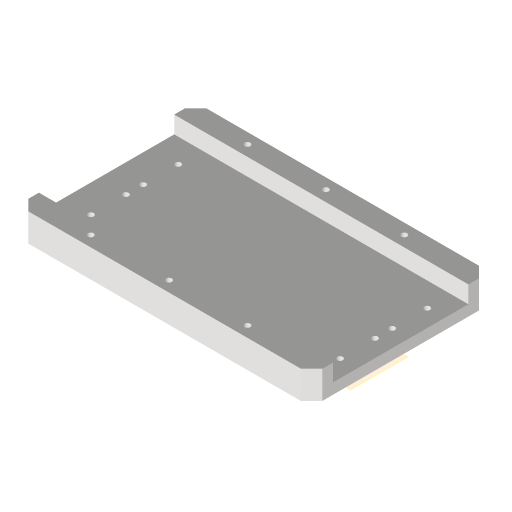
# Autodesk Inventor part: 60_Planktoscope_Wallboxmoutingplate
Saved by Autodesk Inventor 2024.1 (Build 281209000, 209)
## iProperties
Created: 2024-03-15
Part Number: 60_Planktoscope_Wallboxmoutingplate
Material: Generisch
Document SubType Name: Modeling
Designer: diederichbenedict
Density: 1 g/cm^3
Appearance: Vorgabe
Author: diederichbenedict
Autodesk Inventor part; units mm, degrees
ref_plane "YZ Plane" through (0, 0, 0) normal (1, 0, 0) x (0, 1, 0)
ref_plane "XZ Plane" through (0, 0, 0) normal (0, 1, 0) x (-1, 0, 0)
ref_plane "XY Plane" through (0, 0, 0) normal (0, 0, 1) x (1, 0, 0)
ref_plane "Arbeitsebene1" through (0, -48.6, 0) normal (0, 0, 1) x (1, 0, 0)
sketch "Skizze1" plane through (0, -48.6, 0) normal (0, 0, 1) x (1, 0, 0)
  circle A0 centre (124, 28.3) radius 1.4 projected
  circle A1 centre (124, 44.6) radius 1.4 projected
  circle A2 centre (8, 28.3) radius 1.4 projected
  circle A3 centre (8, 44.6) radius 1.4 projected
  spline S0 degree 2 poles (11.2125, 42.0174) (10.5764, 41.5903) (9.8857, 40.1908) (9.8857, 39.2184) knots 0 0 0 1 2 2 2 construction
  spline S1 degree 2 poles (14.1568, 42.7535) (13.1936, 42.7535) (11.785, 42.3991) (11.2125, 42.0174) knots 0 0 0 1 2 2 2 construction
  line L0 (18.5098, 42.7535) -> (14.1568, 42.7535) construction
  line L1 (18.5098, 31.5395) -> (18.5098, 42.7535) construction
  line L2 (15.6926, 31.5395) -> (18.5098, 31.5395) construction
  line L3 (15.6926, 35.2108) -> (15.6926, 31.5395) construction
  line L4 (14.2205, 35.2108) -> (15.6926, 35.2108) construction
  spline S2 degree 2 poles (12.2303, 35.5834) (12.6483, 35.4108) (13.6207, 35.2108) (14.2205, 35.2108) knots 0 0 0 1 2 2 2 construction
  spline S3 degree 2 poles (10.849, 36.5467) (11.1307, 36.2468) (11.8213, 35.7561) (12.2303, 35.5834) knots 0 0 0 1 2 2 2 construction
  spline S4 degree 2 poles (9.8857, 39.2184) (9.8857, 38.4369) (10.3855, 37.0193) (10.849, 36.5467) knots 0 0 0 1 2 2 2 construction
  spline S5 degree 2 poles (25.6162, 42.9898) (23.0899, 42.9898) (20.1819, 39.8637) (20.1819, 37.1465) knots 0 0 0 1 2 2 2 construction
  spline S6 degree 2 poles (31.0415, 37.1465) (31.0415, 39.8455) (28.1516, 42.9898) (25.6162, 42.9898) knots 0 0 0 1 2 2 2 construction
  spline S7 degree 2 poles (25.6162, 31.3032) (28.1516, 31.3032) (31.0415, 34.4566) (31.0415, 37.1465) knots 0 0 0 1 2 2 2 construction
  spline S8 degree 2 poles (20.1819, 37.1465) (20.1819, 34.4202) (23.0899, 31.3032) (25.6162, 31.3032) knots 0 0 0 1 2 2 2 construction
  spline S9 degree 2 poles (37.4936, 42.9898) (34.9673, 42.9898) (32.0593, 39.8637) (32.0593, 37.1465) knots 0 0 0 1 2 2 2 construction
  spline S10 degree 2 poles (42.9188, 37.1465) (42.9188, 39.8455) (40.029, 42.9898) (37.4936, 42.9898) knots 0 0 0 1 2 2 2 construction
  spline S11 degree 2 poles (37.4936, 31.3032) (40.029, 31.3032) (42.9188, 34.4566) (42.9188, 37.1465) knots 0 0 0 1 2 2 2 construction
  spline S12 degree 2 poles (32.0593, 37.1465) (32.0593, 34.4202) (34.9673, 31.3032) (37.4936, 31.3032) knots 0 0 0 1 2 2 2 construction
  line L5 (56.2684, 35.8379) -> (53.1696, 31.5395) construction
  line L6 (53.2059, 40) -> (56.2684, 35.8379) construction
  line L7 (56.2321, 40) -> (53.2059, 40) construction
  line L8 (57.8224, 37.619) -> (56.2321, 40) construction
  line L9 (59.4036, 40) -> (57.8224, 37.619) construction
  line L10 (62.4934, 40) -> (59.4036, 40) construction
  line L11 (59.4309, 35.7743) -> (62.4934, 40) construction
  line L12 (62.5479, 31.5395) -> (59.4309, 35.7743) construction
  line L13 (59.5217, 31.5395) -> (62.5479, 31.5395) construction
  line L14 (57.8678, 33.9659) -> (59.5217, 31.5395) construction
  line L15 (56.2593, 31.5395) -> (57.8678, 33.9659) construction
  line L16 (53.1696, 31.5395) -> (56.2593, 31.5395) construction
  spline S13 degree 2 poles (72.6805, 31.6667) (73.1712, 31.5031) (74.0072, 31.3396) (74.6797, 31.3396) knots 0 0 0 1 2 2 2 construction
  spline S14 degree 2 poles (71.1901, 32.3028) (71.5627, 32.1302) (72.217, 31.8121) (72.6805, 31.6667) knots 0 0 0 1 2 2 2 construction
  line L17 (71.1901, 34.084) -> (71.1901, 32.3028) construction
  line L18 (71.2992, 34.084) -> (71.1901, 34.084) construction
  spline S15 degree 2 poles (72.4896, 33.1843) (72.0807, 33.4206) (71.4718, 33.9113) (71.2992, 34.084) knots 0 0 0 1 2 2 2 construction
  spline S16 degree 2 poles (74.6615, 32.63) (74.0163, 32.63) (72.9167, 32.9481) (72.4896, 33.1843) knots 0 0 0 1 2 2 2 construction
  spline S17 degree 2 poles (77.1061, 33.7478) (76.6335, 33.1934) (75.3704, 32.63) (74.6615, 32.63) knots 0 0 0 1 2 2 2 construction
  spline S18 degree 2 poles (78.1421, 37.1374) (78.1421, 35.9833) (77.5877, 34.3203) (77.1061, 33.7478) knots 0 0 0 1 2 2 2 construction
  spline S19 degree 2 poles (77.1424, 40.527) (77.615, 39.9545) (78.1421, 38.2188) (78.1421, 37.1374) knots 0 0 0 1 2 2 2 construction
  spline S20 degree 2 poles (74.6615, 41.6812) (75.3795, 41.6812) (76.6608, 41.0905) (77.1424, 40.527) knots 0 0 0 1 2 2 2 construction
  spline S21 degree 2 poles (72.5714, 41.145) (72.9985, 41.3813) (74.0072, 41.6812) (74.6615, 41.6812) knots 0 0 0 1 2 2 2 construction
  spline S22 degree 2 poles (71.3083, 40.209) (71.5082, 40.3907) (72.1261, 40.8996) (72.5714, 41.145) knots 0 0 0 1 2 2 2 construction
  line L19 (71.1901, 40.209) -> (71.3083, 40.209) construction
  line L20 (71.1901, 42.0083) -> (71.1901, 40.209) construction
  spline S23 degree 2 poles (72.6805, 42.6626) (72.317, 42.5445) (71.5627, 42.2082) (71.1901, 42.0083) knots 0 0 0 1 2 2 2 construction
  spline S24 degree 2 poles (74.6525, 42.9534) (74.089, 42.9534) (73.0985, 42.7898) (72.6805, 42.6626) knots 0 0 0 1 2 2 2 construction
  spline S25 degree 2 poles (78.2966, 41.4085) (77.6241, 42.1628) (75.7884, 42.9534) (74.6525, 42.9534) knots 0 0 0 1 2 2 2 construction
  spline S26 degree 2 poles (79.696, 37.1374) (79.696, 38.546) (78.9781, 40.6361) (78.2966, 41.4085) knots 0 0 0 1 2 2 2 construction
  spline S27 degree 2 poles (78.2875, 32.8117) (78.9599, 33.5387) (79.696, 35.7198) (79.696, 37.1374) knots 0 0 0 1 2 2 2 construction
  spline S28 degree 2 poles (74.6797, 31.3396) (75.7702, 31.3396) (77.615, 32.0757) (78.2875, 32.8117) knots 0 0 0 1 2 2 2 construction
  line L21 (91.2735, 37.0011) -> (91.2735, 31.5395) construction
  spline S29 degree 2 poles (93.9089, 40.1908) (92.673, 40.1908) (91.2735, 38.5551) (91.2735, 37.0011) knots 0 0 0 1 2 2 2 construction
  spline S30 degree 2 poles (96.4625, 39.0185) (95.8264, 39.591) (94.5996, 40.1908) (93.9089, 40.1908) knots 0 0 0 1 2 2 2 construction
  line L22 (96.4625, 39.9545) -> (96.4625, 39.0185) construction
  line L23 (97.8802, 39.9545) -> (96.4625, 39.9545) construction
  line L24 (97.8802, 31.5395) -> (97.8802, 39.9545) construction
  line L25 (96.4625, 31.5395) -> (97.8802, 31.5395) construction
  line L26 (96.4625, 37.8281) -> (96.4625, 31.5395) construction
  spline S31 degree 2 poles (94.2815, 38.8459) (94.8086, 38.8459) (95.9263, 38.2824) (96.4625, 37.8281) knots 0 0 0 1 2 2 2 construction
  spline S32 degree 2 poles (92.9638, 38.2188) (93.1365, 38.5369) (93.7544, 38.8459) (94.2815, 38.8459) knots 0 0 0 1 2 2 2 construction
  spline S33 degree 2 poles (92.6912, 36.3377) (92.6912, 36.9193) (92.8002, 37.9189) (92.9638, 38.2188) knots 0 0 0 1 2 2 2 construction
  line L27 (92.6912, 31.5395) -> (92.6912, 36.3377) construction
  line L28 (91.2735, 31.5395) -> (92.6912, 31.5395) construction
  spline S34 degree 2 poles (100.7518, 31.5849) (101.1608, 31.4668) (101.8332, 31.3487) (102.3421, 31.3487) knots 0 0 0 1 2 2 2 construction
  spline S35 degree 2 poles (99.4705, 32.0575) (99.7158, 31.9575) (100.461, 31.6667) (100.7518, 31.5849) knots 0 0 0 1 2 2 2 construction
  line L29 (99.4705, 33.6024) -> (99.4705, 32.0575) construction
  line L30 (99.5523, 33.6024) -> (99.4705, 33.6024) construction
  spline S36 degree 2 poles (100.6337, 32.9571) (100.252, 33.1389) (99.7249, 33.457) (99.5523, 33.6024) knots 0 0 0 1 2 2 2 construction
  spline S37 degree 2 poles (102.3603, 32.5846) (101.8968, 32.5846) (100.9972, 32.7936) (100.6337, 32.9571) knots 0 0 0 1 2 2 2 construction
  spline S38 degree 2 poles (105.1411, 35.6016) (105.1411, 34.1385) (103.6689, 32.5846) (102.3603, 32.5846) knots 0 0 0 1 2 2 2 construction
  line L31 (99.316, 35.6016) -> (105.1411, 35.6016) construction
  line L32 (99.316, 36.3741) -> (99.316, 35.6016) construction
  spline S39 degree 2 poles (100.252, 39.2548) (99.7976, 38.7732) (99.316, 37.3828) (99.316, 36.3741) knots 0 0 0 1 2 2 2 construction
  spline S40 degree 2 poles (102.6875, 40.1908) (101.9059, 40.1908) (100.6973, 39.7364) (100.252, 39.2548) knots 0 0 0 1 2 2 2 construction
  spline S41 degree 2 poles (106.5769, 35.7016) (106.5769, 37.7554) (104.4232, 40.1908) (102.6875, 40.1908) knots 0 0 0 1 2 2 2 construction
  spline S42 degree 2 poles (102.3421, 31.3487) (104.3596, 31.3487) (106.5769, 33.6114) (106.5769, 35.7016) knots 0 0 0 1 2 2 2 construction
  spline S43 degree 2 poles (110.53, 40.1908) (109.0851, 40.1908) (107.4675, 37.9008) (107.4675, 35.9742) knots 0 0 0 1 2 2 2 construction
  spline S44 degree 2 poles (113.1018, 39.073) (112.5747, 39.5547) (111.2843, 40.1908) (110.53, 40.1908) knots 0 0 0 1 2 2 2 construction
  line L33 (113.1018, 39.9545) -> (113.1018, 39.073) construction
  line L34 (114.5194, 39.9545) -> (113.1018, 39.9545) construction
  line L35 (114.5194, 28.4406) -> (114.5194, 39.9545) construction
  line L36 (113.1018, 28.4406) -> (114.5194, 28.4406) construction
  line L37 (113.1018, 31.9666) -> (113.1018, 28.4406) construction
  spline S45 degree 2 poles (111.0116, 31.3759) (111.6387, 31.3759) (112.6019, 31.6667) (113.1018, 31.9666) knots 0 0 0 1 2 2 2 construction
  spline S46 degree 2 poles (107.4675, 35.9742) (107.4675, 33.8659) (109.4758, 31.3759) (111.0116, 31.3759) knots 0 0 0 1 2 2 2 construction
  spline S47 degree 2 poles (119.7266, 40.1908) (118.0181, 40.1908) (115.9734, 37.8644) (115.9734, 35.747) knots 0 0 0 1 2 2 2 construction
  spline S48 degree 2 poles (123.4888, 35.747) (123.4888, 37.8553) (121.4168, 40.1908) (119.7266, 40.1908) knots 0 0 0 1 2 2 2 construction
  spline S49 degree 2 poles (119.7266, 31.3032) (121.4805, 31.3032) (123.4888, 33.6932) (123.4888, 35.747) knots 0 0 0 1 2 2 2 construction
  spline S50 degree 2 poles (115.9734, 35.747) (115.9734, 33.6205) (118.0181, 31.3032) (119.7266, 31.3032) knots 0 0 0 1 2 2 2 construction
  spline S51 degree 2 poles (82.2678, 32.3392) (82.804, 31.8121) (84.2216, 31.3032) (85.2576, 31.3032) knots 0 0 0 1 2 2 2 construction
  spline S52 degree 2 poles (81.1955, 35.7561) (81.1955, 34.5838) (81.668, 32.9117) (82.2678, 32.3392) knots 0 0 0 1 2 2 2 construction
  line L38 (81.1955, 42.7535) -> (81.1955, 35.7561) construction
  line L39 (82.6858, 42.7535) -> (81.1955, 42.7535) construction
  line L40 (82.6858, 35.7198) -> (82.6858, 42.7535) construction
  spline S53 degree 2 poles (83.1675, 33.4933) (82.8858, 33.9204) (82.6858, 34.9655) (82.6858, 35.7198) knots 0 0 0 1 2 2 2 construction
  spline S54 degree 2 poles (85.2576, 32.5755) (84.5579, 32.5755) (83.4674, 33.0389) (83.1675, 33.4933) knots 0 0 0 1 2 2 2 construction
  spline S55 degree 2 poles (87.3386, 33.4933) (87.0388, 33.0389) (86.0028, 32.5755) (85.2576, 32.5755) knots 0 0 0 1 2 2 2 construction
  spline S56 degree 2 poles (87.8203, 35.7561) (87.8203, 34.9746) (87.6204, 33.9204) (87.3386, 33.4933) knots 0 0 0 1 2 2 2 construction
  line L41 (87.8203, 42.7535) -> (87.8203, 35.7561) construction
  line L42 (89.3106, 42.7535) -> (87.8203, 42.7535) construction
  line L43 (89.3106, 35.7561) -> (89.3106, 42.7535) construction
  spline S57 degree 2 poles (88.2383, 32.3392) (88.829, 32.9208) (89.3106, 34.5565) (89.3106, 35.7561) knots 0 0 0 1 2 2 2 construction
  spline S58 degree 2 poles (85.2576, 31.3032) (86.2481, 31.3032) (87.7203, 31.8212) (88.2383, 32.3392) knots 0 0 0 1 2 2 2 construction
  line L44 (63.2022, 32.839) -> (63.2022, 31.5395) construction
  line L45 (68.7092, 32.839) -> (63.2022, 32.839) construction
  spline S59 degree 2 poles (65.7467, 35.747) (66.4555, 34.9746) (68.1912, 33.3206) (68.7092, 32.839) knots 0 0 0 1 2 2 2 construction
  spline S60 degree 2 poles (64.2472, 37.6645) (64.5199, 37.1738) (65.3105, 36.2105) (65.7467, 35.747) knots 0 0 0 1 2 2 2 construction
  spline S61 degree 2 poles (63.6656, 39.9091) (63.6656, 39.2457) (63.9746, 38.137) (64.2472, 37.6645) knots 0 0 0 1 2 2 2 construction
  spline S62 degree 2 poles (67.0099, 42.9898) (65.4377, 42.9898) (63.6656, 41.3268) (63.6656, 39.9091) knots 0 0 0 1 2 2 2 construction
  spline S63 degree 2 poles (69.8815, 42.3173) (69.418, 42.5445) (67.755, 42.9898) (67.0099, 42.9898) knots 0 0 0 1 2 2 2 construction
  line L46 (69.8815, 40.7179) -> (69.8815, 42.3173) construction
  line L47 (69.7997, 40.7179) -> (69.8815, 40.7179) construction
  spline S64 degree 2 poles (68.7092, 41.3358) (69.0273, 41.2086) (69.618, 40.8451) (69.7997, 40.7179) knots 0 0 0 1 2 2 2 construction
  spline S65 degree 2 poles (67.1189, 41.6903) (67.5188, 41.6903) (68.3366, 41.4903) (68.7092, 41.3358) knots 0 0 0 1 2 2 2 construction
  spline S66 degree 2 poles (65.7467, 41.2359) (66.0102, 41.4631) (66.7009, 41.6903) (67.1189, 41.6903) knots 0 0 0 1 2 2 2 construction
  spline S67 degree 2 poles (65.1924, 39.8273) (65.1924, 40.2999) (65.4832, 41.0087) (65.7467, 41.2359) knots 0 0 0 1 2 2 2 construction
  spline S68 degree 2 poles (67.4097, 35.8288) (66.1284, 37.2374) (65.1924, 38.9276) (65.1924, 39.8273) knots 0 0 0 1 2 2 2 construction
  spline S69 degree 2 poles (70.1178, 33.1298) (69.3726, 33.8295) (68.0458, 35.1291) (67.4097, 35.8288) knots 0 0 0 1 2 2 2 construction
  line L48 (70.1178, 31.5395) -> (70.1178, 33.1298) construction
  line L49 (63.2022, 31.5395) -> (70.1178, 31.5395) construction
  spline S70 degree 2 poles (43.7095, 35.0473) (43.7095, 33.3752) (46.3357, 31.3396) (48.5713, 31.3396) knots 0 0 0 1 2 2 2 construction
  spline S71 degree 2 poles (46.0086, 38.0552) (44.8454, 37.6281) (43.7095, 36.2105) (43.7095, 35.0473) knots 0 0 0 1 2 2 2 construction
  spline S72 degree 2 poles (48.2169, 38.6368) (47.6534, 38.5096) (46.6084, 38.2643) (46.0086, 38.0552) knots 0 0 0 1 2 2 2 construction
  spline S73 degree 2 poles (49.6981, 39.7728) (49.6981, 39.3366) (49.0893, 38.8368) (48.2169, 38.6368) knots 0 0 0 1 2 2 2 construction
  spline S74 degree 2 poles (49.0529, 40.6543) (49.3165, 40.5361) (49.6981, 40.0636) (49.6981, 39.7728) knots 0 0 0 1 2 2 2 construction
  spline S75 degree 2 poles (47.7716, 40.9087) (48.1442, 40.9087) (48.7258, 40.7997) (49.0529, 40.6543) knots 0 0 0 1 2 2 2 construction
  spline S76 degree 2 poles (44.4001, 39.6365) (45.0271, 40.1726) (46.8265, 40.9087) (47.7716, 40.9087) knots 0 0 0 1 2 2 2 construction
  line L50 (44.1547, 39.6365) -> (44.4001, 39.6365) construction
  line L51 (44.1547, 42.1992) -> (44.1547, 39.6365) construction
  spline S77 degree 2 poles (47.917, 42.9534) (46.9173, 42.9534) (44.9363, 42.5445) (44.1547, 42.1992) knots 0 0 0 1 2 2 2 construction
  spline S78 degree 2 poles (52.5789, 39.4275) (52.5789, 40.9996) (49.9162, 42.9534) (47.917, 42.9534) knots 0 0 0 1 2 2 2 construction
  spline S79 degree 2 poles (50.1525, 36.2559) (51.452, 36.7103) (52.5789, 38.2643) (52.5789, 39.4275) knots 0 0 0 1 2 2 2 construction
  spline S80 degree 2 poles (47.708, 35.638) (48.2805, 35.7925) (49.58, 36.056) (50.1525, 36.2559) knots 0 0 0 1 2 2 2 construction
  spline S81 degree 2 poles (46.5902, 34.5656) (46.5902, 34.9927) (47.2536, 35.5198) (47.708, 35.638) knots 0 0 0 1 2 2 2 construction
  spline S82 degree 2 poles (47.2899, 33.6024) (46.9991, 33.7296) (46.5902, 34.193) (46.5902, 34.5656) knots 0 0 0 1 2 2 2 construction
  spline S83 degree 2 poles (48.5622, 33.3843) (48.3168, 33.3843) (47.5262, 33.4933) (47.2899, 33.6024) knots 0 0 0 1 2 2 2 construction
  spline S84 degree 2 poles (52.388, 34.8746) (51.5429, 34.1567) (49.5164, 33.3843) (48.5622, 33.3843) knots 0 0 0 1 2 2 2 construction
  line L52 (52.6425, 34.8746) -> (52.388, 34.8746) construction
  line L53 (52.6425, 32.2029) -> (52.6425, 34.8746) construction
  spline S85 degree 2 poles (48.5713, 31.3396) (49.8617, 31.3396) (51.8064, 31.8394) (52.6425, 32.2029) knots 0 0 0 1 2 2 2 construction
  line L54 (128, 24.3) -> (128, 48.6) projected
  line L55 (4, 48.6) -> (128, 48.6) projected
  line L56 (4, 48.6) -> (4, 24.3) projected
  line L57 (4, 24.3) -> (128, 24.3) construction
  circle A4 centre (124, 20.3) radius 1.4 projected
  circle A5 centre (124, 4) radius 1.4 projected
  circle A6 centre (8, 20.3) radius 1.4 projected
  circle A7 centre (8, 4) radius 1.4 projected
  spline S86 degree 2 poles (11.2125, 6.5826) (10.5764, 7.0097) (9.8857, 8.4092) (9.8857, 9.3816) knots 0 0 0 1 2 2 2 construction
  spline S87 degree 2 poles (9.8857, 9.3816) (9.8857, 10.1631) (10.3855, 11.5807) (10.849, 12.0533) knots 0 0 0 1 2 2 2 construction
  spline S88 degree 2 poles (10.849, 12.0533) (11.1307, 12.3532) (11.8213, 12.8439) (12.2303, 13.0166) knots 0 0 0 1 2 2 2 construction
  spline S89 degree 2 poles (12.2303, 13.0166) (12.6483, 13.1892) (13.6207, 13.3892) (14.2205, 13.3892) knots 0 0 0 1 2 2 2 construction
  line L58 (14.2205, 13.3892) -> (15.6926, 13.3892) construction
  line L59 (15.6926, 13.3892) -> (15.6926, 17.0605) construction
  line L60 (15.6926, 17.0605) -> (18.5098, 17.0605) construction
  line L61 (18.5098, 17.0605) -> (18.5098, 5.8465) construction
  line L62 (18.5098, 5.8465) -> (14.1568, 5.8465) construction
  spline S90 degree 2 poles (14.1568, 5.8465) (13.1936, 5.8465) (11.785, 6.2009) (11.2125, 6.5826) knots 0 0 0 1 2 2 2 construction
  spline S91 degree 2 poles (25.6162, 5.6102) (23.0899, 5.6102) (20.1819, 8.7363) (20.1819, 11.4535) knots 0 0 0 1 2 2 2 construction
  spline S92 degree 2 poles (20.1819, 11.4535) (20.1819, 14.1798) (23.0899, 17.2968) (25.6162, 17.2968) knots 0 0 0 1 2 2 2 construction
  spline S93 degree 2 poles (25.6162, 17.2968) (28.1516, 17.2968) (31.0415, 14.1434) (31.0415, 11.4535) knots 0 0 0 1 2 2 2 construction
  spline S94 degree 2 poles (31.0415, 11.4535) (31.0415, 8.7545) (28.1516, 5.6102) (25.6162, 5.6102) knots 0 0 0 1 2 2 2 construction
  spline S95 degree 2 poles (37.4936, 5.6102) (34.9673, 5.6102) (32.0593, 8.7363) (32.0593, 11.4535) knots 0 0 0 1 2 2 2 construction
  spline S96 degree 2 poles (32.0593, 11.4535) (32.0593, 14.1798) (34.9673, 17.2968) (37.4936, 17.2968) knots 0 0 0 1 2 2 2 construction
  spline S97 degree 2 poles (37.4936, 17.2968) (40.029, 17.2968) (42.9188, 14.1434) (42.9188, 11.4535) knots 0 0 0 1 2 2 2 construction
  spline S98 degree 2 poles (42.9188, 11.4535) (42.9188, 8.7545) (40.029, 5.6102) (37.4936, 5.6102) knots 0 0 0 1 2 2 2 construction
  line L63 (56.2684, 12.7621) -> (53.1696, 17.0605) construction
  line L64 (53.1696, 17.0605) -> (56.2593, 17.0605) construction
  line L65 (56.2593, 17.0605) -> (57.8678, 14.6341) construction
  line L66 (57.8678, 14.6341) -> (59.5217, 17.0605) construction
  line L67 (59.5217, 17.0605) -> (62.5479, 17.0605) construction
  line L68 (62.5479, 17.0605) -> (59.4309, 12.8257) construction
  line L69 (59.4309, 12.8257) -> (62.4934, 8.6) construction
  line L70 (62.4934, 8.6) -> (59.4036, 8.6) construction
  line L71 (59.4036, 8.6) -> (57.8224, 10.981) construction
  line L72 (57.8224, 10.981) -> (56.2321, 8.6) construction
  line L73 (56.2321, 8.6) -> (53.2059, 8.6) construction
  line L74 (53.2059, 8.6) -> (56.2684, 12.7621) construction
  spline S99 degree 2 poles (72.6805, 16.9333) (73.1712, 17.0969) (74.0072, 17.2604) (74.6797, 17.2604) knots 0 0 0 1 2 2 2 construction
  spline S100 degree 2 poles (74.6797, 17.2604) (75.7702, 17.2604) (77.615, 16.5243) (78.2875, 15.7883) knots 0 0 0 1 2 2 2 construction
  spline S101 degree 2 poles (78.2875, 15.7883) (78.9599, 15.0613) (79.696, 12.8802) (79.696, 11.4626) knots 0 0 0 1 2 2 2 construction
  spline S102 degree 2 poles (79.696, 11.4626) (79.696, 10.054) (78.9781, 7.9639) (78.2966, 7.1915) knots 0 0 0 1 2 2 2 construction
  spline S103 degree 2 poles (78.2966, 7.1915) (77.6241, 6.4372) (75.7884, 5.6466) (74.6525, 5.6466) knots 0 0 0 1 2 2 2 construction
  spline S104 degree 2 poles (74.6525, 5.6466) (74.089, 5.6466) (73.0985, 5.8102) (72.6805, 5.9374) knots 0 0 0 1 2 2 2 construction
  spline S105 degree 2 poles (72.6805, 5.9374) (72.317, 6.0555) (71.5627, 6.3918) (71.1901, 6.5917) knots 0 0 0 1 2 2 2 construction
  line L75 (71.1901, 6.5917) -> (71.1901, 8.391) construction
  line L76 (71.1901, 8.391) -> (71.3083, 8.391) construction
  spline S106 degree 2 poles (71.3083, 8.391) (71.5082, 8.2093) (72.1261, 7.7004) (72.5714, 7.455) knots 0 0 0 1 2 2 2 construction
  spline S107 degree 2 poles (72.5714, 7.455) (72.9985, 7.2187) (74.0072, 6.9188) (74.6615, 6.9188) knots 0 0 0 1 2 2 2 construction
  spline S108 degree 2 poles (74.6615, 6.9188) (75.3795, 6.9188) (76.6608, 7.5095) (77.1424, 8.073) knots 0 0 0 1 2 2 2 construction
  spline S109 degree 2 poles (77.1424, 8.073) (77.615, 8.6455) (78.1421, 10.3812) (78.1421, 11.4626) knots 0 0 0 1 2 2 2 construction
  spline S110 degree 2 poles (78.1421, 11.4626) (78.1421, 12.6167) (77.5877, 14.2797) (77.1061, 14.8522) knots 0 0 0 1 2 2 2 construction
  spline S111 degree 2 poles (77.1061, 14.8522) (76.6335, 15.4066) (75.3704, 15.97) (74.6615, 15.97) knots 0 0 0 1 2 2 2 construction
  spline S112 degree 2 poles (74.6615, 15.97) (74.0163, 15.97) (72.9167, 15.6519) (72.4896, 15.4157) knots 0 0 0 1 2 2 2 construction
  spline S113 degree 2 poles (72.4896, 15.4157) (72.0807, 15.1794) (71.4718, 14.6887) (71.2992, 14.516) knots 0 0 0 1 2 2 2 construction
  line L77 (71.2992, 14.516) -> (71.1901, 14.516) construction
  line L78 (71.1901, 14.516) -> (71.1901, 16.2972) construction
  spline S114 degree 2 poles (71.1901, 16.2972) (71.5627, 16.4698) (72.217, 16.7879) (72.6805, 16.9333) knots 0 0 0 1 2 2 2 construction
  line L79 (91.2735, 11.5989) -> (91.2735, 17.0605) construction
  line L80 (91.2735, 17.0605) -> (92.6912, 17.0605) construction
  line L81 (92.6912, 17.0605) -> (92.6912, 12.2623) construction
  spline S115 degree 2 poles (92.6912, 12.2623) (92.6912, 11.6807) (92.8002, 10.6811) (92.9638, 10.3812) knots 0 0 0 1 2 2 2 construction
  spline S116 degree 2 poles (92.9638, 10.3812) (93.1365, 10.0631) (93.7544, 9.7541) (94.2815, 9.7541) knots 0 0 0 1 2 2 2 construction
  spline S117 degree 2 poles (94.2815, 9.7541) (94.8086, 9.7541) (95.9263, 10.3176) (96.4625, 10.7719) knots 0 0 0 1 2 2 2 construction
  line L82 (96.4625, 10.7719) -> (96.4625, 17.0605) construction
  line L83 (96.4625, 17.0605) -> (97.8802, 17.0605) construction
  line L84 (97.8802, 17.0605) -> (97.8802, 8.6455) construction
  line L85 (97.8802, 8.6455) -> (96.4625, 8.6455) construction
  line L86 (96.4625, 8.6455) -> (96.4625, 9.5815) construction
  spline S118 degree 2 poles (96.4625, 9.5815) (95.8264, 9.009) (94.5996, 8.4092) (93.9089, 8.4092) knots 0 0 0 1 2 2 2 construction
  spline S119 degree 2 poles (93.9089, 8.4092) (92.673, 8.4092) (91.2735, 10.0449) (91.2735, 11.5989) knots 0 0 0 1 2 2 2 construction
  spline S120 degree 2 poles (100.7518, 17.0151) (101.1608, 17.1332) (101.8332, 17.2513) (102.3421, 17.2513) knots 0 0 0 1 2 2 2 construction
  spline S121 degree 2 poles (102.3421, 17.2513) (104.3596, 17.2513) (106.5769, 14.9886) (106.5769, 12.8984) knots 0 0 0 1 2 2 2 construction
  spline S122 degree 2 poles (106.5769, 12.8984) (106.5769, 10.8446) (104.4232, 8.4092) (102.6875, 8.4092) knots 0 0 0 1 2 2 2 construction
  spline S123 degree 2 poles (102.6875, 8.4092) (101.9059, 8.4092) (100.6973, 8.8636) (100.252, 9.3452) knots 0 0 0 1 2 2 2 construction
  spline S124 degree 2 poles (100.252, 9.3452) (99.7976, 9.8268) (99.316, 11.2172) (99.316, 12.2259) knots 0 0 0 1 2 2 2 construction
  line L87 (99.316, 12.2259) -> (99.316, 12.9984) construction
  line L88 (99.316, 12.9984) -> (105.1411, 12.9984) construction
  spline S125 degree 2 poles (105.1411, 12.9984) (105.1411, 14.4615) (103.6689, 16.0154) (102.3603, 16.0154) knots 0 0 0 1 2 2 2 construction
  spline S126 degree 2 poles (102.3603, 16.0154) (101.8968, 16.0154) (100.9972, 15.8064) (100.6337, 15.6429) knots 0 0 0 1 2 2 2 construction
  spline S127 degree 2 poles (100.6337, 15.6429) (100.252, 15.4611) (99.7249, 15.143) (99.5523, 14.9976) knots 0 0 0 1 2 2 2 construction
  line L89 (99.5523, 14.9976) -> (99.4705, 14.9976) construction
  line L90 (99.4705, 14.9976) -> (99.4705, 16.5425) construction
  spline S128 degree 2 poles (99.4705, 16.5425) (99.7158, 16.6425) (100.461, 16.9333) (100.7518, 17.0151) knots 0 0 0 1 2 2 2 construction
  spline S129 degree 2 poles (110.53, 8.4092) (109.0851, 8.4092) (107.4675, 10.6992) (107.4675, 12.6258) knots 0 0 0 1 2 2 2 construction
  spline S130 degree 2 poles (107.4675, 12.6258) (107.4675, 14.7341) (109.4758, 17.2241) (111.0116, 17.2241) knots 0 0 0 1 2 2 2 construction
  spline S131 degree 2 poles (111.0116, 17.2241) (111.6387, 17.2241) (112.6019, 16.9333) (113.1018, 16.6334) knots 0 0 0 1 2 2 2 construction
  line L91 (113.1018, 16.6334) -> (113.1018, 20.1594) construction
  line L92 (113.1018, 20.1594) -> (114.5194, 20.1594) construction
  line L93 (114.5194, 20.1594) -> (114.5194, 8.6455) construction
  line L94 (114.5194, 8.6455) -> (113.1018, 8.6455) construction
  line L95 (113.1018, 8.6455) -> (113.1018, 9.527) construction
  spline S132 degree 2 poles (113.1018, 9.527) (112.5747, 9.0453) (111.2843, 8.4092) (110.53, 8.4092) knots 0 0 0 1 2 2 2 construction
  spline S133 degree 2 poles (119.7266, 8.4092) (118.0181, 8.4092) (115.9734, 10.7356) (115.9734, 12.853) knots 0 0 0 1 2 2 2 construction
  spline S134 degree 2 poles (115.9734, 12.853) (115.9734, 14.9795) (118.0181, 17.2968) (119.7266, 17.2968) knots 0 0 0 1 2 2 2 construction
  spline S135 degree 2 poles (119.7266, 17.2968) (121.4805, 17.2968) (123.4888, 14.9068) (123.4888, 12.853) knots 0 0 0 1 2 2 2 construction
  spline S136 degree 2 poles (123.4888, 12.853) (123.4888, 10.7447) (121.4168, 8.4092) (119.7266, 8.4092) knots 0 0 0 1 2 2 2 construction
  spline S137 degree 2 poles (82.2678, 16.2608) (82.804, 16.7879) (84.2216, 17.2968) (85.2576, 17.2968) knots 0 0 0 1 2 2 2 construction
  spline S138 degree 2 poles (85.2576, 17.2968) (86.2481, 17.2968) (87.7203, 16.7788) (88.2383, 16.2608) knots 0 0 0 1 2 2 2 construction
  spline S139 degree 2 poles (88.2383, 16.2608) (88.829, 15.6792) (89.3106, 14.0435) (89.3106, 12.8439) knots 0 0 0 1 2 2 2 construction
  line L96 (89.3106, 12.8439) -> (89.3106, 5.8465) construction
  line L97 (89.3106, 5.8465) -> (87.8203, 5.8465) construction
  line L98 (87.8203, 5.8465) -> (87.8203, 12.8439) construction
  spline S140 degree 2 poles (87.8203, 12.8439) (87.8203, 13.6254) (87.6204, 14.6796) (87.3386, 15.1067) knots 0 0 0 1 2 2 2 construction
  spline S141 degree 2 poles (87.3386, 15.1067) (87.0388, 15.5611) (86.0028, 16.0245) (85.2576, 16.0245) knots 0 0 0 1 2 2 2 construction
  spline S142 degree 2 poles (85.2576, 16.0245) (84.5579, 16.0245) (83.4674, 15.5611) (83.1675, 15.1067) knots 0 0 0 1 2 2 2 construction
  spline S143 degree 2 poles (83.1675, 15.1067) (82.8858, 14.6796) (82.6858, 13.6345) (82.6858, 12.8802) knots 0 0 0 1 2 2 2 construction
  line L99 (82.6858, 12.8802) -> (82.6858, 5.8465) construction
  line L100 (82.6858, 5.8465) -> (81.1955, 5.8465) construction
  line L101 (81.1955, 5.8465) -> (81.1955, 12.8439) construction
  spline S144 degree 2 poles (81.1955, 12.8439) (81.1955, 14.0162) (81.668, 15.6883) (82.2678, 16.2608) knots 0 0 0 1 2 2 2 construction
  line L102 (63.2022, 15.761) -> (63.2022, 17.0605) construction
  line L103 (63.2022, 17.0605) -> (70.1178, 17.0605) construction
  line L104 (70.1178, 17.0605) -> (70.1178, 15.4702) construction
  spline S145 degree 2 poles (70.1178, 15.4702) (69.3726, 14.7705) (68.0458, 13.4709) (67.4097, 12.7712) knots 0 0 0 1 2 2 2 construction
  spline S146 degree 2 poles (67.4097, 12.7712) (66.1284, 11.3626) (65.1924, 9.6724) (65.1924, 8.7727) knots 0 0 0 1 2 2 2 construction
  spline S147 degree 2 poles (65.1924, 8.7727) (65.1924, 8.3001) (65.4832, 7.5913) (65.7467, 7.3641) knots 0 0 0 1 2 2 2 construction
  spline S148 degree 2 poles (65.7467, 7.3641) (66.0102, 7.1369) (66.7009, 6.9097) (67.1189, 6.9097) knots 0 0 0 1 2 2 2 construction
  spline S149 degree 2 poles (67.1189, 6.9097) (67.5188, 6.9097) (68.3366, 7.1097) (68.7092, 7.2642) knots 0 0 0 1 2 2 2 construction
  spline S150 degree 2 poles (68.7092, 7.2642) (69.0273, 7.3914) (69.618, 7.7549) (69.7997, 7.8821) knots 0 0 0 1 2 2 2 construction
  line L105 (69.7997, 7.8821) -> (69.8815, 7.8821) construction
  line L106 (69.8815, 7.8821) -> (69.8815, 6.2827) construction
  spline S151 degree 2 poles (69.8815, 6.2827) (69.418, 6.0555) (67.755, 5.6102) (67.0099, 5.6102) knots 0 0 0 1 2 2 2 construction
  spline S152 degree 2 poles (67.0099, 5.6102) (65.4377, 5.6102) (63.6656, 7.2732) (63.6656, 8.6909) knots 0 0 0 1 2 2 2 construction
  spline S153 degree 2 poles (63.6656, 8.6909) (63.6656, 9.3543) (63.9746, 10.463) (64.2472, 10.9355) knots 0 0 0 1 2 2 2 construction
  spline S154 degree 2 poles (64.2472, 10.9355) (64.5199, 11.4262) (65.3105, 12.3895) (65.7467, 12.853) knots 0 0 0 1 2 2 2 construction
  spline S155 degree 2 poles (65.7467, 12.853) (66.4555, 13.6254) (68.1912, 15.2794) (68.7092, 15.761) knots 0 0 0 1 2 2 2 construction
  line L107 (68.7092, 15.761) -> (63.2022, 15.761) construction
  spline S156 degree 2 poles (43.7095, 13.5527) (43.7095, 15.2248) (46.3357, 17.2604) (48.5713, 17.2604) knots 0 0 0 1 2 2 2 construction
  spline S157 degree 2 poles (48.5713, 17.2604) (49.8617, 17.2604) (51.8064, 16.7606) (52.6425, 16.3971) knots 0 0 0 1 2 2 2 construction
  line L108 (52.6425, 16.3971) -> (52.6425, 13.7254) construction
  line L109 (52.6425, 13.7254) -> (52.388, 13.7254) construction
  spline S158 degree 2 poles (52.388, 13.7254) (51.5429, 14.4433) (49.5164, 15.2157) (48.5622, 15.2157) knots 0 0 0 1 2 2 2 construction
  spline S159 degree 2 poles (48.5622, 15.2157) (48.3168, 15.2157) (47.5262, 15.1067) (47.2899, 14.9976) knots 0 0 0 1 2 2 2 construction
  spline S160 degree 2 poles (47.2899, 14.9976) (46.9991, 14.8704) (46.5902, 14.407) (46.5902, 14.0344) knots 0 0 0 1 2 2 2 construction
  spline S161 degree 2 poles (46.5902, 14.0344) (46.5902, 13.6073) (47.2536, 13.0802) (47.708, 12.962) knots 0 0 0 1 2 2 2 construction
  spline S162 degree 2 poles (47.708, 12.962) (48.2805, 12.8075) (49.58, 12.544) (50.1525, 12.3441) knots 0 0 0 1 2 2 2 construction
  spline S163 degree 2 poles (50.1525, 12.3441) (51.452, 11.8897) (52.5789, 10.3357) (52.5789, 9.1725) knots 0 0 0 1 2 2 2 construction
  spline S164 degree 2 poles (52.5789, 9.1725) (52.5789, 7.6004) (49.9162, 5.6466) (47.917, 5.6466) knots 0 0 0 1 2 2 2 construction
  spline S165 degree 2 poles (47.917, 5.6466) (46.9173, 5.6466) (44.9363, 6.0555) (44.1547, 6.4008) knots 0 0 0 1 2 2 2 construction
  line L110 (44.1547, 6.4008) -> (44.1547, 8.9635) construction
  line L111 (44.1547, 8.9635) -> (44.4001, 8.9635) construction
  spline S166 degree 2 poles (44.4001, 8.9635) (45.0271, 8.4274) (46.8265, 7.6913) (47.7716, 7.6913) knots 0 0 0 1 2 2 2 construction
  spline S167 degree 2 poles (47.7716, 7.6913) (48.1442, 7.6913) (48.7258, 7.8003) (49.0529, 7.9457) knots 0 0 0 1 2 2 2 construction
  spline S168 degree 2 poles (49.0529, 7.9457) (49.3165, 8.0639) (49.6981, 8.5364) (49.6981, 8.8272) knots 0 0 0 1 2 2 2 construction
  spline S169 degree 2 poles (49.6981, 8.8272) (49.6981, 9.2634) (49.0893, 9.7632) (48.2169, 9.9632) knots 0 0 0 1 2 2 2 construction
  spline S170 degree 2 poles (48.2169, 9.9632) (47.6534, 10.0904) (46.6084, 10.3357) (46.0086, 10.5448) knots 0 0 0 1 2 2 2 construction
  spline S171 degree 2 poles (46.0086, 10.5448) (44.8454, 10.9719) (43.7095, 12.3895) (43.7095, 13.5527) knots 0 0 0 1 2 2 2 construction
  line L112 (128, 24.3) -> (128, 0) projected
  line L113 (4, 24.3) -> (128, 24.3) construction
  line L114 (4, 0) -> (4, 24.3) projected
  line L115 (4, 0) -> (128, 0) construction
  line L116 (-5, 2) -> (-5, 46.6) projected
  line L117 (132, 48.6) -> (132, 24.3) projected
  line L118 (132, 48.6) -> (-5, 48.6)
  line L119 (-5, 48.6) -> (-5, 0)
  line L120 (-5, 0) -> (132, 0)
  line L121 (132, 0) -> (132, 48.6)
  circle A8 centre (24.0952, 60.8) radius 5 projected
  circle A9 centre (24.0952, 60.8) radius 1.4 projected
  circle A10 centre (60.5952, 60.8) radius 5 projected
  circle A11 centre (97.0952, 60.8) radius 5 projected
  circle A12 centre (24.0952, -12.2) radius 1.4 projected
  circle A13 centre (60.5952, -12.2) radius 1.4 projected
  circle A14 centre (97.0952, -12.2) radius 1.4 projected
  circle A15 centre (97.0952, 60.8) radius 1.4 projected
  circle A16 centre (97.0952, -12.2) radius 5 projected
  line L122 (-5, 65.8) -> (132, 65.8)
  line L123 (132, 65.8) -> (132, -17.2)
  line L124 (132, -17.2) -> (-5, -17.2)
  line L125 (-5, -17.2) -> (-5, 65.8)
  circle A17 centre (60.5952, 60.8) radius 1.4
  point P0 (0, 48.6)
  point P1 (60.5952, 65.8)
  point P2 (24.0952, 65.8)
  point P3 (-5, 48.6)
  dimension "d2" = 2.8
  constraints: 16 end point, 4 parallel, 2 horizontal, 2 perpendicular, 1 centre point, 1 coincident
  measures "d2" diameter of A17
extrude "Extrusion1" add sketch "Skizze1" along normal blind 5 contours L112 L120 L114 L56 L55 L54 | L54 L118 L117 L121 L120 L112 | A11 | A10 | A8 | L55 L118 L125 L122 L123 | A16 | L120 L123 L124 L125 | L56 L114 L120 L119 L116 L118 | A9
chamfer "Fasen1" distance 5 angle 45 4 edges at (-5, 17.2, 2.5) (132, 17.2, 2.5) (-5, -65.8, 2.5) (132, -65.8, 2.5)
sketch "Skizze2" plane through (0, -48.6, 0) normal (0, 0, -1) x (-1, 0, 0)
  line L0 (-127, -17.2) -> (-132, -12.2) projected
  line L1 (0, -17.2) -> (-127, -17.2) projected
  line L2 (5, -12.2) -> (0, -17.2) projected
  line L3 (5, 60.8) -> (5, -12.2) projected
  line L4 (0, 65.8) -> (5, 60.8) projected
  line L5 (-127, 65.8) -> (0, 65.8) projected
  line L6 (-132, 60.8) -> (-127, 65.8) projected
  line L7 (-132, -12.2) -> (-132, 60.8) projected
  circle A0 centre (-8, 20.3) radius 1.4 projected
  circle A1 centre (-124, 4) radius 1.4 projected
  circle A2 centre (-124, 20.3) radius 1.4 projected
  circle A3 centre (-8, 44.6) radius 1.4 projected
  circle A4 centre (-8, 28.3) radius 1.4 projected
  circle A5 centre (-124, 44.6) radius 1.4 projected
  circle A6 centre (-124, 28.3) radius 1.4 projected
  circle A7 centre (-8, 4) radius 1.4 projected
  circle A8 centre (-24.0952, -12.2) radius 1.4 projected
  circle A9 centre (-60.5952, -12.2) radius 1.4 projected
  circle A10 centre (-97.0952, -12.2) radius 1.4 projected
  circle A11 centre (-97.0952, 60.8) radius 1.4 projected
  circle A12 centre (-60.5952, 60.8) radius 1.4 projected
  line L8 (-103.75, 48.6) -> (-4, 48.6) projected
  line L9 (-103.75, 0) -> (-4, 0) projected
  line L10 (5, 49.1) -> (-132, 49.1)
  line L11 (-132, 49.1) -> (-132, -0.5)
  line L12 (-132, -0.5) -> (5, -0.5)
  line L13 (5, -0.5) -> (5, 49.1)
  point P0 (0, 48.6)
  point P1 (5, -0.5)
  dimension "d6" = 0.5
  dimension "d7" = 0.5
  constraints: 8 end point, 2 parallel, 2 point on line, 1 horizontal, 1 perpendicular
  measures "d6" distance between parallel lines of L8 L10
  measures "d7" distance between parallel lines of L9 L12
extrude "Extrusion2" [suppressed]
sketch "Skizze3" plane through (0, -48.6, 5) normal (0, 0, 1) x (1, 0, 0)
  line L0 (132, -12.2) -> (127, -17.2) projected
  line L1 (132, -12.2) -> (132, 60.8) projected
  line L2 (127, 65.8) -> (132, 60.8) projected
  line L3 (127, 65.8) -> (0, 65.8) projected
  line L4 (-5, 60.8) -> (0, 65.8) projected
  line L5 (-5, 60.8) -> (-5, -12.2) projected
  line L6 (0, -17.2) -> (-5, -12.2) projected
  line L7 (0, -17.2) -> (127, -17.2) projected
  circle A0 centre (8, 20.3) radius 1.4 projected
  circle A1 centre (124, 4) radius 1.4 projected
  circle A2 centre (124, 20.3) radius 1.4 projected
  circle A3 centre (8, 44.6) radius 1.4 projected
  circle A4 centre (8, 28.3) radius 1.4 projected
  circle A5 centre (124, 44.6) radius 1.4 projected
  circle A6 centre (124, 28.3) radius 1.4 projected
  circle A7 centre (8, 4) radius 1.4 projected
  circle A8 centre (24.0952, -12.2) radius 1.4 projected
  circle A9 centre (60.5952, -12.2) radius 1.4 projected
  circle A10 centre (97.0952, -12.2) radius 1.4 projected
  circle A11 centre (97.0952, 60.8) radius 1.4 projected
  circle A12 centre (60.5952, 60.8) radius 1.4 projected
  circle A13 centre (24.0952, 60.8) radius 1.4 projected
  line L8 (-5, -17.2) -> (132, -17.2)
  line L9 (132, -17.2) -> (132, -7.2)
  line L10 (132, -7.2) -> (-5, -7.2)
  line L11 (-5, -7.2) -> (-5, -17.2)
  line L12 (132, 60.8) -> (132, 49.1) projected
  line L13 (-5, 65.8) -> (132, 65.8)
  line L14 (132, 65.8) -> (132, 55.8)
  line L15 (132, 55.8) -> (-5, 55.8)
  line L16 (-5, 55.8) -> (-5, 65.8)
  point P0 (0, 48.6)
  point P1 (-5, 55.8)
  point P2 (-5, -7.2)
  dimension "d10" = 10
  dimension "d11" = 10
  constraints: 16 end point, 4 parallel, 3 point on line, 2 horizontal, 2 perpendicular
  measures "d10" distance of L9.end L8.end
  measures "d11" distance of L13.end L14.end
extrude "Extrusion3" add sketch "Skizze3" along normal blind 8 contours L0 L7 L6 L5 L10 L1 | L15 L5 L4 L3 L2 L1
